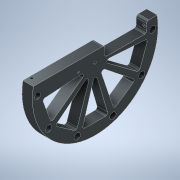
# Autodesk Inventor part: Capstondisc
Saved by Autodesk Inventor 2022 (Build 260153000, 153)
## iProperties
Created: 2022-03-10
Part Number: Capstondisc
Material: Generisch
Document SubType Name: Modeling
Designer: 123St
Density: 1 g/cm^3
Appearance: Eisen - Grau
Author: 123St
Autodesk Inventor part; units mm, degrees
ref_plane "YZ Plane" through (0, 0, 0) normal (1, 0, 0) x (0, 1, 0)
ref_plane "XZ Plane" through (0, 0, 0) normal (0, 1, 0) x (-1, 0, 0)
ref_plane "XY Plane" through (0, 0, 0) normal (0, 0, 1) x (1, 0, 0)
sketch "Skizze1" plane through (0, 0, 0) normal (1, 0, 0) x (0, 1, 0)
  arc A0 (10, 59.1608) -> (10, -59.1608) centre (0, 0) ccw
  line L0 (10, 59.1608) -> (10, -9.1608)
  line L1 (10, -59.1608) -> (10, -49.1608)
  line L2 (10, -9.1608) -> (0, -9.1608)
  line L3 (0, -9.1608) -> (0, -49.1608)
  line L4 (0, -49.1608) -> (10, -49.1608)
  circle A1 centre (0, 55) radius 3
  circle A2 centre (-32.3282, 44.4959) radius 3
  circle A3 centre (-52.3081, 16.9959) radius 3
  circle A4 centre (-52.3081, -16.9959) radius 3
  circle A5 centre (-32.3282, -44.4959) radius 3
  circle A6 centre (0, -55) radius 3
  circle A7 centre (0, 0) radius 1.25
  line L5 (-7, 0) -> (-49.1993, 12.5)
  line L6 (-49.1993, 12.5) -> (-49.1993, -12.5)
  line L7 (-49.1993, -12.5) -> (-7, 0)
  line L8 (-74, 0) -> (24, 0) projected
  line L9 (-33.132, -38.459) -> (-5.7341, -4.015)
  line L10 (-5.7341, -4.015) -> (-47.4714, -17.9802)
  line L11 (-47.4714, -17.9802) -> (-33.132, -38.459)
  line L12 (-5.081, -50.5075) -> (-2.3941, -6.5778)
  line L13 (-2.3941, -6.5778) -> (-28.5733, -41.957)
  line L14 (-28.5733, -41.957) -> (-5.081, -50.5075)
  line L15 (-33.132, 38.459) -> (-5.7341, 4.015)
  line L16 (-5.7341, 4.015) -> (-47.4714, 17.9802)
  line L17 (-47.4714, 17.9802) -> (-33.132, 38.459)
  line L18 (-5.081, 50.5075) -> (-2.3941, 6.5778)
  line L19 (-2.3941, 6.5778) -> (-28.5733, 41.957)
  line L20 (-28.5733, 41.957) -> (-5.081, 50.5075)
  dimension "d0" = 120
  dimension "d1" = 40
  dimension "d2" = 10
  dimension "d3" = 10
  dimension "d4" = 10
  dimension "d5" = 10
  dimension "d6" = 55
  dimension "d7" = 0
  dimension "d8" = 6
  dimension "d11" = 180
  dimension "d13" = 2.5
  dimension "d19" = 33
  dimension "d20" = 12.5
  dimension "d22" = 0
  dimension "d23" = 7
  dimension "d26" = 70
  dimension "d34" = 25
  constraints: 40 end point, 8 centre point, 6 symmetric about line, 3 vertical, 2 coincident, 2 perpendicular, 2 point on circle, 1 horizontal, 24 other
  measures "d0" diameter of A0
  measures "d1" distance of L2.end L3.end
  measures "d2" distance of L1.start L1.end
  measures "d3" distance from line of point (0, 0) L0
  measures "d4" distance from line of point (0, 0) L1
  measures "d5" distance of L3.end L1.end
  measures "d6" distance of A1.centre point (0, 0)
  measures "d7" horizontal distance of point (0, 0) A1.centre
  measures "d8" diameter of A1
  measures "d13" diameter of A7
  measures "d19" angle of L7 L5
  measures "d20" distance from line of L5.end L8
  measures "d22" distance from line of L8 L5.start
  measures "d23" distance of point (0, 0) L5.start
  measures "d34" distance of L5.end L6.end
extrude "Extrusion1" add sketch "Skizze1" along normal blind 10 contours L0 L8 A7 L5 L6 A0 | L8 L6 L7 A7 L0 L2 L3 L4 L1 A0
fillet "Rundung1" radius 2 15 edges at (5, -5.081, -50.5075) (5, -28.5733, -41.957) (5, -33.132, -38.459) (5, -47.4714, -17.9802) (5, -49.1993, -12.5) (5, -49.1993, 12.5) (5, -33.132, 38.459) (5, -47.4714, 17.9802) (5, -28.5733, 41.957) (5, -5.081, 50.5075) (5, -2.3941, 6.5778) (5, -5.7341, 4.015) (5, -7, 0) (5, -5.7341, -4.015) (5, -2.3941, -6.5778)
fillet "Rundung2" radius 2 4 edges at (5, 10, -9.1608) (5, 0, -9.1608) (5, 0, -49.1608) (5, 10, -49.1608)
sketch "Skizze2" plane through (10, 0, 0) normal (1, 0, 0) x (0, 0, -1)
  circle A0 centre (-16, 0) radius 0.75
  point P0 (0, 0)
  dimension "d30" = 1.5
  dimension "d31" = 16
  constraints: 1 centre point
  measures "d30" diameter of A0
  measures "d31" distance of point (0, 0) A0.centre
extrude "Extrusion2" cut sketch "Skizze2" against normal blind 10
sketch "Skizze3" plane through (0, 2, -49.1608) normal (0, 0, 1) x (1, 0, 0)
  circle A0 centre (7.5, 3) radius 1.25
  line L0 (10, 6) -> (10, 0) projected
  line L1 (0, 6) -> (10, 6) projected
  point P0 (0, -2)
  dimension "d35" = 2.5
  dimension "d36" = 2.5
  dimension "d37" = 3
  constraints: 1 centre point
  measures "d35" diameter of A0
  measures "d36" distance from line of L0 A0.centre
  measures "d37" distance from line of L1 A0.centre
extrude "Extrusion3" cut sketch "Skizze3" against normal blind 12
sketch "Skizze4" plane through (0, 10, 59.1608) normal (0, 1, 0) x (1, 0, 0)
  circle A0 centre (2.5, 6) radius 1.25
  line L0 (0, 66.3216) -> (0, 0) projected
  line L1 (0, 0) -> (10, 0) projected
  point P0 (0, 59.1608)
  dimension "d40" = 2.5
  dimension "d41" = 2.5
  dimension "d42" = 6
  constraints: 1 centre point
  measures "d40" diameter of A0
  measures "d41" distance from line of L0 A0.centre
  measures "d42" distance from line of L1 A0.centre
extrude "Extrusion4" cut sketch "Skizze4" against normal blind 10
equation "\"d20\" = 0.5 * d34"
